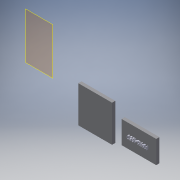
# Autodesk Inventor part: IC_names
Saved by Autodesk Inventor 2016 (Build 200138000, 138)
## iProperties
Created: 2016-04-08
Part Number: IC_names
Material: Generic
Document SubType Name: Modeling
Designer: Paschalis
Density: 1 g/cm^3
Appearance: Default
Author: Paschalis
Autodesk Inventor part; units mm, degrees
ref_plane "YZ Plane" through (0, 0, 0) normal (1, 0, 0) x (0, 1, 0)
ref_plane "XZ Plane" through (0, 0, 0) normal (0, 1, 0) x (-1, 0, 0)
ref_plane "XY Plane" through (0, 0, 0) normal (0, 0, 1) x (1, 0, 0)
ref_plane "Work Plane1" through (-32.0167, 10.0112, 0) normal (0, 0, 1) x (0, 1, 0)
sketch "Sketch1" plane through (-32.0167, 10.0112, 0) normal (0, 0, 1) x (0, 1, 0)
  line L0 (-6.4884, -37.4012) -> (-6.4884, -26.6323) projected
  line L1 (-6.4884, -26.6323) -> (-13.534, -26.6323) projected
  line L2 (-13.534, -26.6323) -> (-13.534, -37.4012) projected
  line L3 (-13.534, -37.4012) -> (-6.4884, -37.4012) projected
  line L4 (-3.5941, -13.1572) -> (-14.9225, -13.1572) projected
  line L5 (-14.9225, -13.1572) -> (-14.9225, -23.6728) projected
  line L6 (-14.9225, -23.6728) -> (-3.5941, -23.6728) projected
  line L7 (-3.5941, -23.6728) -> (-3.5941, -13.1572) projected
  line L8 (17.6149, -8.1534) -> (17.6149, -17.2466) projected
  line L9 (17.6149, -17.2466) -> (26.7081, -17.2466) projected
  line L10 (26.7081, -17.2466) -> (26.7081, -8.1534) projected
  line L11 (26.7081, -8.1534) -> (17.6149, -8.1534) projected
  line L12 (14.8209, 36.449) -> (6.6421, 36.449) projected
  line L13 (6.6421, 36.449) -> (6.6421, 25.8572) projected
  line L14 (6.6421, 25.8572) -> (14.8209, 25.8572) projected
  line L15 (14.8209, 25.8572) -> (14.8209, 36.449) projected
  line L16 (-1.5621, 51.6636) -> (-1.5621, 48.6664) projected
  line L17 (-1.5621, 48.6664) -> (1.5113, 48.6664) projected
  line L18 (1.5113, 48.6664) -> (1.5113, 51.6636) projected
  line L19 (1.5113, 51.6636) -> (-1.5621, 51.6636) projected
  line L20 (23.6601, 51.054) -> (20.6629, 51.054) projected
  line L21 (20.6629, 51.054) -> (20.6629, 47.9298) projected
  line L22 (20.6629, 47.9298) -> (23.6601, 47.9298) projected
  line L23 (23.6601, 47.9298) -> (23.6601, 51.054) projected
  point P0 (-10.0112, -32.0167)
extrude "Extrusion1" add sketch "Sketch1" along normal blind 1 contours L3 L2 L1 L0 | L7 L6 L5 L4
sketch "Sketch2" plane through (-32.0167, 10.0112, 1) normal (0, 0, 1) x (1, 0, 0)
  line L0 (35.0354, -10.5466) -> (28.7851, -10.5466) construction
  line L1 (28.7851, -10.5466) -> (28.7851, -7.5923) construction
  line L2 (28.7851, -7.5923) -> (35.0354, -7.5923) construction
  line L3 (35.0354, -7.5923) -> (35.0354, -10.5466) construction
  line L4 (34.0857, -9.5335) -> (34.2174, -9.5335)
  line L5 (34.2174, -9.5335) -> (34.2174, -10.3869)
  line L6 (34.2174, -10.3869) -> (34.4759, -9.8065)
  line L7 (34.4759, -9.8065) -> (34.5561, -9.8065)
  line L8 (34.5561, -9.8065) -> (34.8122, -10.3869)
  line L9 (34.8122, -10.3869) -> (34.8122, -9.5335)
  line L10 (34.8122, -9.5335) -> (34.935, -9.5335)
  line L11 (34.935, -9.5335) -> (34.935, -10.5241)
  line L12 (34.935, -10.5241) -> (34.7552, -10.5241)
  line L13 (34.7552, -10.5241) -> (34.508, -9.9726)
  line L14 (34.508, -9.9726) -> (34.2688, -10.5241)
  line L15 (34.2688, -10.5241) -> (34.0857, -10.5241)
  line L16 (34.0857, -10.5241) -> (34.0857, -9.5335)
  line L17 (33.9918, -9.5335) -> (33.6579, -10.5241)
  line L18 (33.6579, -10.5241) -> (33.4957, -10.5241)
  line L19 (33.4957, -10.5241) -> (33.1618, -9.5335)
  line L20 (33.1618, -9.5335) -> (33.3006, -9.5335)
  line L21 (33.3006, -9.5335) -> (33.3905, -9.8105)
  line L22 (33.3905, -9.8105) -> (33.7686, -9.8105)
  line L23 (33.7686, -9.8105) -> (33.8585, -9.5335)
  line L24 (33.8585, -9.5335) -> (33.9918, -9.5335)
  line L25 (33.4267, -9.9229) -> (33.58, -10.3893)
  line L26 (33.58, -10.3893) -> (33.7325, -9.9229)
  line L27 (33.7325, -9.9229) -> (33.4267, -9.9229)
  line L28 (32.3831, -9.5335) -> (32.534, -9.5335)
  line L29 (32.534, -9.5335) -> (32.7748, -9.9285)
  line L30 (32.7748, -9.9285) -> (33.0205, -9.5335)
  line L31 (33.0205, -9.5335) -> (33.1626, -9.5335)
  line L32 (33.1626, -9.5335) -> (32.8471, -10.0296)
  line L33 (32.8471, -10.0296) -> (33.1529, -10.5241)
  line L34 (33.1529, -10.5241) -> (33.002, -10.5241)
  line L35 (33.002, -10.5241) -> (32.766, -10.1364)
  line L36 (32.766, -10.1364) -> (32.5252, -10.5241)
  line L37 (32.5252, -10.5241) -> (32.3831, -10.5241)
  line L38 (32.3831, -10.5241) -> (32.6929, -10.0361)
  line L39 (32.6929, -10.0361) -> (32.3831, -9.5335)
  line L40 (31.7441, -9.5335) -> (32.2273, -9.5335)
  line L41 (32.2273, -9.5335) -> (32.2273, -9.6347)
  line L42 (32.2273, -9.6347) -> (32.0475, -9.6347)
  line L43 (32.0475, -9.6347) -> (32.0475, -10.2986)
  line L44 (32.0475, -10.2986) -> (32.2273, -10.2986)
  line L45 (32.2273, -10.2986) -> (32.2273, -10.3893)
  spline S0 degree 2 poles (32.2273, -10.3893) (32.1254, -10.3893) (32.0291, -10.4471) (32.0226, -10.5273) knots 0 0 0 1 2 2 2
  line L46 (32.0226, -10.5273) -> (31.9199, -10.5273)
  line L47 (31.9199, -10.5273) -> (31.9199, -9.6347)
  line L48 (31.9199, -9.6347) -> (31.7441, -9.6347)
  line L49 (31.7441, -9.6347) -> (31.7441, -9.5335)
  line L50 (30.9245, -9.8739) -> (31.0425, -9.8739)
  line L51 (31.0425, -9.8739) -> (31.0425, -9.5335)
  line L52 (31.0425, -9.5335) -> (31.1701, -9.5335)
  line L53 (31.1701, -9.5335) -> (31.1701, -9.8739)
  line L54 (31.1701, -9.8739) -> (31.6076, -9.8739)
  line L55 (31.6076, -9.8739) -> (31.6076, -10.0136)
  line L56 (31.6076, -10.0136) -> (31.1645, -10.5241)
  line L57 (31.1645, -10.5241) -> (31.0425, -10.5241)
  line L58 (31.0425, -10.5241) -> (31.0425, -9.9807)
  line L59 (31.0425, -9.9807) -> (30.9245, -9.9807)
  line L60 (30.9245, -9.9807) -> (30.9245, -9.8739)
  line L61 (31.1701, -9.9807) -> (31.1701, -10.3676)
  line L62 (31.1701, -10.3676) -> (31.5033, -9.9807)
  line L63 (31.5033, -9.9807) -> (31.1701, -9.9807)
  spline S1 degree 2 poles (30.5191, -9.5111) (30.5929, -9.5111) (30.7142, -9.5552) (30.7567, -9.5961) knots 0 0 0 1 2 2 2
  spline S2 degree 2 poles (30.7567, -9.5961) (30.7984, -9.6363) (30.8418, -9.7455) (30.8418, -9.8073) knots 0 0 0 1 2 2 2
  spline S3 degree 2 poles (30.8418, -9.8073) (30.8418, -9.8875) (30.7559, -10.0224) (30.674, -10.0625) knots 0 0 0 1 2 2 2
  line L64 (30.674, -10.0625) -> (30.674, -10.0666)
  spline S4 degree 2 poles (30.674, -10.0666) (30.7471, -10.1091) (30.8177, -10.2103) (30.8177, -10.2857) knots 0 0 0 1 2 2 2
  spline S5 degree 2 poles (30.8177, -10.2857) (30.8177, -10.3973) (30.6491, -10.5466) (30.5191, -10.5466) knots 0 0 0 1 2 2 2
  spline S6 degree 2 poles (30.5191, -10.5466) (30.3842, -10.5466) (30.2213, -10.4053) (30.2213, -10.2945) knots 0 0 0 1 2 2 2
  spline S7 degree 2 poles (30.2213, -10.2945) (30.2213, -10.2279) (30.2991, -10.0979) (30.3722, -10.0609) knots 0 0 0 1 2 2 2
  line L65 (30.3722, -10.0609) -> (30.3722, -10.0569)
  spline S8 degree 2 poles (30.3722, -10.0569) (30.2855, -10.0168) (30.1964, -9.9012) (30.1964, -9.8097) knots 0 0 0 1 2 2 2
  spline S9 degree 2 poles (30.1964, -9.8097) (30.1964, -9.6828) (30.381, -9.5111) (30.5191, -9.5111) knots 0 0 0 1 2 2 2
  spline S10 degree 2 poles (30.3328, -9.7968) (30.3328, -9.8578) (30.381, -9.9301) (30.4492, -9.967) knots 0 0 0 1 2 2 2
  spline S11 degree 2 poles (30.4492, -9.967) (30.4717, -9.9799) (30.5472, -10.0096) (30.5945, -10.0288) knots 0 0 0 1 2 2 2
  spline S12 degree 2 poles (30.5945, -10.0288) (30.6491, -9.9927) (30.7077, -9.8851) (30.7077, -9.8169) knots 0 0 0 1 2 2 2
  spline S13 degree 2 poles (30.7077, -9.8169) (30.7077, -9.727) (30.5994, -9.6098) (30.5175, -9.6098) knots 0 0 0 1 2 2 2
  spline S14 degree 2 poles (30.5175, -9.6098) (30.434, -9.6098) (30.3328, -9.7101) (30.3328, -9.7968) knots 0 0 0 1 2 2 2
  spline S15 degree 2 poles (30.3513, -10.2929) (30.3513, -10.3596) (30.4404, -10.4487) (30.5199, -10.4487) knots 0 0 0 1 2 2 2
  spline S16 degree 2 poles (30.5199, -10.4487) (30.5921, -10.4487) (30.6845, -10.3692) (30.6845, -10.301) knots 0 0 0 1 2 2 2
  spline S17 degree 2 poles (30.6845, -10.301) (30.6845, -10.252) (30.6371, -10.1838) (30.5897, -10.1565) knots 0 0 0 1 2 2 2
  spline S18 degree 2 poles (30.5897, -10.1565) (30.5697, -10.1452) (30.4846, -10.1059) (30.45, -10.0947) knots 0 0 0 1 2 2 2
  spline S19 degree 2 poles (30.45, -10.0947) (30.3923, -10.1388) (30.3513, -10.2327) (30.3513, -10.2929) knots 0 0 0 1 2 2 2
  spline S20 degree 2 poles (29.4747, -9.8482) (29.4747, -9.7768) (29.5205, -9.6547) (29.5622, -9.6098) knots 0 0 0 1 2 2 2
  spline S21 degree 2 poles (29.5622, -9.6098) (29.6039, -9.5648) (29.7284, -9.5127) (29.8054, -9.5127) knots 0 0 0 1 2 2 2
  spline S22 degree 2 poles (29.8054, -9.5127) (29.8761, -9.5127) (30.0142, -9.544) (30.0647, -9.5689) knots 0 0 0 1 2 2 2
  line L66 (30.0647, -9.5689) -> (30.0647, -9.7093)
  line L67 (30.0647, -9.7093) -> (30.0551, -9.7093)
  spline S23 degree 2 poles (30.0551, -9.7093) (30.0398, -9.6981) (29.9828, -9.6692) (29.9483, -9.6564) knots 0 0 0 1 2 2 2
  spline S24 degree 2 poles (29.9483, -9.6564) (29.909, -9.6427) (29.844, -9.6275) (29.803, -9.6275) knots 0 0 0 1 2 2 2
  spline S25 degree 2 poles (29.803, -9.6275) (29.7629, -9.6275) (29.6874, -9.6564) (29.6601, -9.6877) knots 0 0 0 1 2 2 2
  spline S26 degree 2 poles (29.6601, -9.6877) (29.6353, -9.7174) (29.6096, -9.796) (29.6096, -9.849) knots 0 0 0 1 2 2 2
  spline S27 degree 2 poles (29.6096, -9.849) (29.6096, -9.902) (29.6385, -9.9694) (29.6658, -9.9919) knots 0 0 0 1 2 2 2
  spline S28 degree 2 poles (29.6658, -9.9919) (29.6939, -10.0168) (29.7773, -10.0377) (29.8279, -10.0377) knots 0 0 0 1 2 2 2
  spline S29 degree 2 poles (29.8279, -10.0377) (29.8825, -10.0377) (29.9909, -10.0208) (30.0238, -10.0136) knots 0 0 0 1 2 2 2
  line L68 (30.0238, -10.0136) -> (30.0238, -10.5241)
  line L69 (30.0238, -10.5241) -> (29.4803, -10.5241)
  line L70 (29.4803, -10.5241) -> (29.4803, -10.4077)
  line L71 (29.4803, -10.4077) -> (29.8961, -10.4077)
  line L72 (29.8961, -10.4077) -> (29.8961, -10.1436)
  spline S30 degree 2 poles (29.8961, -10.1436) (29.8721, -10.1468) (29.8255, -10.1492) (29.8062, -10.1492) knots 0 0 0 1 2 2 2
  spline S31 degree 2 poles (29.8062, -10.1492) (29.73, -10.1492) (29.6248, -10.1244) (29.5767, -10.0874) knots 0 0 0 1 2 2 2
  spline S32 degree 2 poles (29.5767, -10.0874) (29.5277, -10.0505) (29.4747, -9.9381) (29.4747, -9.8482) knots 0 0 0 1 2 2 2
  spline S33 degree 2 poles (28.7153, -10.0288) (28.7153, -9.7623) (28.8702, -9.5127) (29.0316, -9.5127) knots 0 0 0 1 2 2 2
  spline S34 degree 2 poles (29.0316, -9.5127) (29.1953, -9.5127) (29.3487, -9.7671) (29.3487, -10.028) knots 0 0 0 1 2 2 2
  spline S35 degree 2 poles (29.3487, -10.028) (29.3487, -10.2962) (29.1937, -10.5442) (29.0316, -10.5442) knots 0 0 0 1 2 2 2
  spline S36 degree 2 poles (29.0316, -10.5442) (28.8686, -10.5442) (28.7153, -10.2873) (28.7153, -10.0288) knots 0 0 0 1 2 2 2
  spline S37 degree 2 poles (28.8855, -9.727) (28.8662, -9.776) (28.8502, -9.9269) (28.8502, -10.0288) knots 0 0 0 1 2 2 2
  spline S38 degree 2 poles (28.8502, -10.0288) (28.8502, -10.1308) (28.8662, -10.2809) (28.8863, -10.3315) knots 0 0 0 1 2 2 2
  spline S39 degree 2 poles (28.8863, -10.3315) (28.9064, -10.382) (28.9762, -10.4342) (29.0316, -10.4342) knots 0 0 0 1 2 2 2
  spline S40 degree 2 poles (29.0316, -10.4342) (29.087, -10.4342) (29.1584, -10.382) (29.1793, -10.3299) knots 0 0 0 1 2 2 2
  spline S41 degree 2 poles (29.1793, -10.3299) (29.1994, -10.2793) (29.2138, -10.1252) (29.2138, -10.028) knots 0 0 0 1 2 2 2
  spline S42 degree 2 poles (29.2138, -10.028) (29.2138, -9.9237) (29.201, -9.784) (29.1801, -9.7294) knots 0 0 0 1 2 2 2
  spline S43 degree 2 poles (29.1801, -9.7294) (29.1608, -9.678) (29.0894, -9.6226) (29.0316, -9.6226) knots 0 0 0 1 2 2 2
  spline S44 degree 2 poles (29.0316, -9.6226) (28.977, -9.6226) (28.9055, -9.6748) (28.8855, -9.727) knots 0 0 0 1 2 2 2
  point P0 (32.0167, -10.0112)
  constraints: 2 other
emboss "Emboss1" sketch "Sketch2" operation add depth 0.5 direction (0, 0, -1)
body "Solid1"
